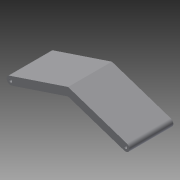
# Autodesk Inventor part: Front Support
Saved by Autodesk Inventor 2015 (Build 190159000, 159)
## iProperties
Created: 2016-08-02
Part Number: Front Support
Material: Generic
Document SubType Name: Modeling
Designer: James Yelland
Density: 1 g/cm^3
Appearance: Default
Author: James Yelland
Autodesk Inventor part; units mm, degrees
ref_plane "YZ Plane" through (0, 0, 0) normal (1, 0, 0) x (0, 1, 0)
ref_plane "XZ Plane" through (0, 0, 0) normal (0, 1, 0) x (-1, 0, 0)
ref_plane "XY Plane" through (0, 0, 0) normal (0, 0, 1) x (1, 0, 0)
sketch "Sketch1" plane through (0, 0, 0) normal (0, 1, 0) x (-1, 0, 0)
  circle A0 centre (59.0549, -74.4145) radius 1.6
  circle A1 centre (-59.0549, -74.4145) radius 1.6
  line L0 (57.79, -78.2092) -> (0, -58.9459)
  line L1 (-57.79, -78.2092) -> (0, -58.9459)
  line L2 (-60.3198, -70.6198) -> (0, -50.5132)
  line L3 (60.3198, -70.6198) -> (0, -50.5132)
  arc A2 (57.79, -78.2092) -> (60.3198, -70.6198) centre (59.0549, -74.4145) ccw
  arc A3 (-60.3198, -70.6198) -> (-57.79, -78.2092) centre (-59.0549, -74.4145) ccw
  constraints: 8 end point, 4 centre point, 4 point on circle, 1 coincident
extrude "Extrusion1" add sketch "Sketch1" along normal blind 45
body "Solid1"
